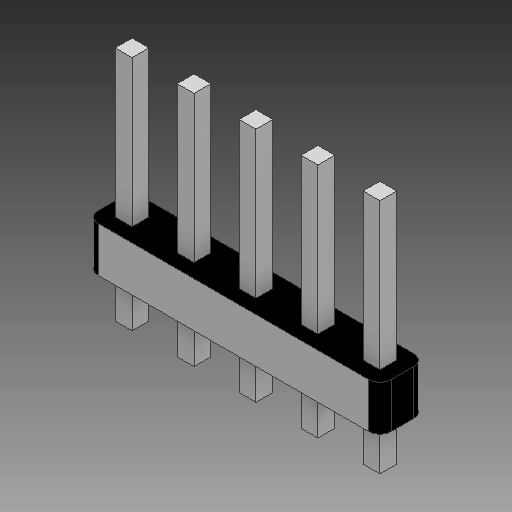
# Autodesk Inventor part: Pinhead 5
Saved by Autodesk Inventor 2018 (Build 220112000, 112)
## iProperties
Created: 2019-03-05
Part Number: Pinhead 5
Material: Generisch
Document SubType Name: Modeling
Designer: RedBots
Density: 1 g/cm^3
Appearance: Vorgabe
Mass: 0.075477 g
Surface Area: 2.37354 cm^2
Volume: 0.075477 cm^3
Author: RedBots
Autodesk Inventor part; units mm, degrees
ref_plane "YZ Plane" through (0, 0, 0) normal (1, 0, 0) x (0, 1, 0)
ref_plane "XZ Plane" through (0, 0, 0) normal (0, 1, 0) x (-1, 0, 0)
ref_plane "XY Plane" through (0, 0, 0) normal (0, 0, 1) x (1, 0, 0)
sketch "Skizze1" plane through (0, 0, 0) normal (0, 0, 1) x (1, 0, 0)
  line L0 (0, 0) -> (13, 0)
  line L1 (13, 0) -> (13, 2)
  line L2 (13, 2) -> (0, 2)
  line L3 (0, 2) -> (0, 0)
  dimension "d0" = 13
  dimension "d1" = 2
  constraints: 8 end point, 2 parallel, 1 horizontal, 1 perpendicular
  measures "d0" distance of L2.end L1.end
  measures "d1" distance of L1.end L0.end
extrude "Extrusion1" add sketch "Skizze1" along normal blind 2
sketch "Skizze2" plane through (0, 0, 2) normal (0, 0, 1) x (1, 0, 0)
  line L0 (6.125, 1.375) -> (6.875, 1.375)
  line L1 (6.875, 1.375) -> (6.875, 0.625)
  line L2 (6.875, 0.625) -> (6.125, 0.625)
  line L3 (6.125, 0.625) -> (6.125, 1.375)
  line L4 (13, 2) -> (0, 2) construction
  line L5 (6.5, 2) -> (6.5, 0) construction
  line L6 (0, 0) -> (13, 0) construction
  line L7 (0, 2) -> (0, 0) construction
  line L8 (0, 1) -> (13, 1) construction
  line L9 (13, 0) -> (13, 2) construction
  line L10 (8.875, 1.375) -> (9.625, 1.375)
  line L11 (8.875, 0.625) -> (8.875, 1.375)
  line L12 (9.625, 0.625) -> (8.875, 0.625)
  line L13 (9.625, 1.375) -> (9.625, 0.625)
  line L14 (11.625, 1.375) -> (12.375, 1.375)
  line L15 (11.625, 0.625) -> (11.625, 1.375)
  line L16 (12.375, 0.625) -> (11.625, 0.625)
  line L17 (12.375, 1.375) -> (12.375, 0.625)
  line L18 (3.375, 1.375) -> (4.125, 1.375)
  line L19 (3.375, 0.625) -> (3.375, 1.375)
  line L20 (4.125, 0.625) -> (3.375, 0.625)
  line L21 (4.125, 1.375) -> (4.125, 0.625)
  line L22 (6.125, 1.375) -> (6.875, 1.375)
  line L23 (6.125, 0.625) -> (6.125, 1.375)
  line L24 (6.875, 0.625) -> (6.125, 0.625)
  line L25 (6.875, 1.375) -> (6.875, 0.625)
  line L26 (8.875, 1.375) -> (9.625, 1.375)
  line L27 (8.875, 0.625) -> (8.875, 1.375)
  line L28 (9.625, 0.625) -> (8.875, 0.625)
  line L29 (9.625, 1.375) -> (9.625, 0.625)
  line L30 (0.625, 1.375) -> (1.375, 1.375)
  line L31 (0.625, 0.625) -> (0.625, 1.375)
  line L32 (1.375, 0.625) -> (0.625, 0.625)
  line L33 (1.375, 1.375) -> (1.375, 0.625)
  line L34 (3.375, 1.375) -> (4.125, 1.375)
  line L35 (3.375, 0.625) -> (3.375, 1.375)
  line L36 (4.125, 0.625) -> (3.375, 0.625)
  line L37 (4.125, 1.375) -> (4.125, 0.625)
  line L38 (6.125, 1.375) -> (6.875, 1.375)
  line L39 (6.125, 0.625) -> (6.125, 1.375)
  line L40 (6.875, 0.625) -> (6.125, 0.625)
  line L41 (6.875, 1.375) -> (6.875, 0.625)
  point P0 (6.5, 1.375)
  point P1 (6.125, 1)
  point P2 (9.25, 1.375)
  point P3 (8.875, 1)
  point P4 (12, 1.375)
  point P5 (11.625, 1)
  point P6 (3.75, 1.375)
  point P7 (3.375, 1)
  point P8 (6.5, 1.375)
  point P9 (6.125, 1)
  point P10 (9.25, 1.375)
  point P11 (8.875, 1)
  point P12 (1, 1.375)
  point P13 (0.625, 1)
  point P14 (3.75, 1.375)
  point P15 (3.375, 1)
  point P16 (6.5, 1.375)
  point P17 (6.125, 1)
  dimension "d4" = 0.75
  dimension "d7" = 2.75
  dimension "d10" = 2.75
  constraints: 76 end point, 6 midpoint, 3 horizontal, 2 parallel, 2 perpendicular, 2 point on line, 80 other
  measures "d4" distance of L1.end L2.end
  measures "d7" distance of L0.start L10.start
  measures "d10" distance of L0.start L18.start
extrude "Extrusion2" add sketch "Skizze2" along normal blind 6.5
sketch "Skizze3" plane through (0, 0, 0) normal (0, 0, -1) x (-1, 0, 0)
  line L0 (-1.375, 1.375) -> (-0.625, 1.375) projected
  line L1 (-0.625, 1.375) -> (-0.625, 0.625) projected
  line L2 (-0.625, 0.625) -> (-1.375, 0.625) projected
  line L3 (-1.375, 0.625) -> (-1.375, 1.375) projected
  line L4 (-4.125, 1.375) -> (-3.375, 1.375) projected
  line L5 (-3.375, 1.375) -> (-3.375, 0.625) projected
  line L6 (-3.375, 0.625) -> (-4.125, 0.625) projected
  line L7 (-4.125, 0.625) -> (-4.125, 1.375) projected
  line L8 (-6.875, 1.375) -> (-6.125, 1.375) projected
  line L9 (-6.125, 1.375) -> (-6.125, 0.625) projected
  line L10 (-6.125, 0.625) -> (-6.875, 0.625) projected
  line L11 (-6.875, 0.625) -> (-6.875, 1.375) projected
  line L12 (-9.625, 0.625) -> (-9.625, 1.375) projected
  line L13 (-9.625, 1.375) -> (-8.875, 1.375) projected
  line L14 (-8.875, 1.375) -> (-8.875, 0.625) projected
  line L15 (-8.875, 0.625) -> (-9.625, 0.625) projected
  line L16 (-9.625, 0.625) -> (-9.625, 1.375) projected
  line L17 (-12.375, 1.375) -> (-11.625, 1.375) projected
  line L18 (-11.625, 1.375) -> (-11.625, 0.625) projected
  line L19 (-11.625, 0.625) -> (-12.375, 0.625) projected
  line L20 (-12.375, 0.625) -> (-12.375, 1.375) projected
  point P0 (0, 0)
extrude "Extrusion3" add sketch "Skizze3" along normal blind 2
fillet "Rundung1" radius 0.5 4 edges at (0, 0, 1) (0, 2, 1) (13, 0, 1) (13, 2, 1)
